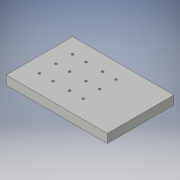
# Autodesk Inventor part: panel
Saved by Autodesk Inventor 2016 (Build 200138000, 138)
## iProperties
Created: 2016-07-20
Part Number: panel
Material: Generic
Document SubType Name: Modeling
Designer: Zuhra Abdurashidova
Density: 1 g/cm^3
Appearance: Default
Author: Zuhra Abdurashidova
Autodesk Inventor part; units mm, degrees
ref_plane "YZ Plane" through (0, 0, 0) normal (1, 0, 0) x (0, 1, 0)
ref_plane "XZ Plane" through (0, 0, 0) normal (0, 1, 0) x (-1, 0, 0)
ref_plane "XY Plane" through (0, 0, 0) normal (0, 0, 1) x (1, 0, 0)
sketch "Sketch1" plane through (0, 0, 0) normal (0, 1, 0) x (-1, 0, 0)
  line L0 (0, 0) -> (-350, 0)
  line L1 (-350, 0) -> (-350, -230)
  line L2 (-350, -230) -> (0, -230)
  line L3 (0, -230) -> (0, 0)
  line L4 (-50, -178) -> (-50, -175)
  arc A0 (-50, -175) -> (-50, -178) centre (-53.1623, -176.5) ccw
  line L5 (-50, -121) -> (-50, -118)
  arc A1 (-50, -118) -> (-50, -121) centre (-53.1623, -119.5) ccw
  line L6 (-50, -64) -> (-50, -61)
  arc A2 (-50, -61) -> (-50, -64) centre (-53.1623, -62.5) ccw
  line L7 (-97, -178) -> (-97, -175)
  arc A3 (-97, -175) -> (-97, -178) centre (-100.1623, -176.5) ccw
  line L8 (-97, -121) -> (-97, -118)
  arc A4 (-97, -118) -> (-97, -121) centre (-100.1623, -119.5) ccw
  line L9 (-97, -64) -> (-97, -61)
  arc A5 (-97, -61) -> (-97, -64) centre (-100.1623, -62.5) ccw
  line L10 (-201, -64) -> (-201, -61)
  line L11 (-201, -121) -> (-201, -118)
  line L12 (-201, -178) -> (-201, -175)
  arc A6 (-201, -61) -> (-201, -64) centre (-204.1623, -62.5) ccw
  arc A7 (-201, -118) -> (-201, -121) centre (-204.1623, -119.5) ccw
  arc A8 (-201, -175) -> (-201, -178) centre (-204.1623, -176.5) ccw
  arc A9 (-154, -61) -> (-154, -64) centre (-157.1623, -62.5) ccw
  arc A10 (-154, -118) -> (-154, -121) centre (-157.1623, -119.5) ccw
  line L13 (-154, -121) -> (-154, -118)
  line L14 (-154, -178) -> (-154, -175)
  arc A11 (-154, -175) -> (-154, -178) centre (-157.1623, -176.5) ccw
  line L15 (-154, -64) -> (-154, -61)
  dimension "d0" = 350
  dimension "d1" = 230
  dimension "d107" = 3.5
  dimension "d109" = 3
  dimension "d110" = 50
  dimension "d111" = 53.5
  dimension "d114" = 57
  dimension "d121" = 47
  dimension "d128" = 104
  constraints: 32 end point, 24 point on circle, 12 centre point, 3 horizontal, 2 parallel, 2 vertical, 1 perpendicular, 55 other
  measures "d0" distance of L1.end L2.end
  measures "d1" distance of L0.end L1.end
  measures "d107" radius of A0
  measures "d109" distance of L4.start L4.end
  measures "d110" distance between parallel lines of L3 L4
  measures "d111" distance from line of L2 A0.centre
  measures "d114" distance of L4.start L5.start
  measures "d121" distance of L4.start L7.start
  measures "d128" distance of L9.start L10.start
extrude "Extrusion2" add sketch "Sketch1" along normal blind 30
body "Solid2"
